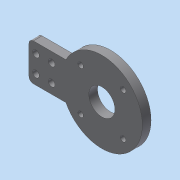
# Autodesk Inventor part: motormount3_B
Saved by Autodesk Inventor 2017 (Build 210142000, 142)
## iProperties
Created: 2015-12-27
Part Number: motormount3_B
Material: Generic
Document SubType Name: Modeling
Designer: JoshuaYuan
Density: 1 g/cm^3
Appearance: Default
Author: JoshuaYuan
Autodesk Inventor part; units mm, degrees
ref_plane "YZ Plane" through (0, 0, 0) normal (1, 0, 0) x (0, 1, 0)
ref_plane "XZ Plane" through (0, 0, 0) normal (0, 1, 0) x (-1, 0, 0)
ref_plane "XY Plane" through (0, 0, 0) normal (0, 0, 1) x (1, 0, 0)
sketch "Sketch1" plane through (0, 0, 0) normal (0, 0, 1) x (1, 0, 0)
  line L0 (-17.3159, 0) -> (99.2924, 0) projected
  line L1 (0, -41.3) -> (0, 41.3) projected
  circle A0 centre (53.1341, 0) radius 29.5
  line L2 (26.924, 13.5382) -> (3.175, 13.5382)
  line L3 (0, 10.3632) -> (0, -10.3632)
  line L4 (3.175, -13.5382) -> (26.924, -13.5382)
  arc A1 (3.175, 13.5382) -> (0, 10.3632) centre (3.175, 10.3632) ccw
  arc A2 (0, -10.3632) -> (3.175, -13.5382) centre (3.175, -10.3632) ccw
  circle A3 centre (5.08, 6.35) radius 2.413
  circle A4 centre (16.51, 6.35) radius 2.413
  circle A5 centre (5.08, -6.35) radius 2.413
  circle A6 centre (16.51, -6.35) radius 2.413
  circle A7 centre (37.6341, 15.5) radius 2
  circle A8 centre (68.6341, 15.5) radius 2
  circle A9 centre (68.6341, -15.5) radius 2
  circle A10 centre (37.6341, -15.5) radius 2
  line L5 (73.9937, 20.8597) -> (32.2744, -20.8597) construction
  line L6 (32.2744, 20.8597) -> (73.9937, -20.8597) construction
  circle A11 centre (53.1341, 0) radius 9.525
  point P0 (0, 0)
  point P1 (0, -13.5382)
  dimension "d0" = 59
  dimension "d2" = 3.175
  dimension "d9" = 20.7264
  dimension "d10" = 4.826
  dimension "d15" = 11.43
  dimension "d18" = 12.7
  dimension "d21" = 4
  dimension "d23" = 4
  dimension "d24" = 4
  dimension "d25" = 4
  dimension "d26" = 45
  dimension "d45" = 19.05
  dimension "d48" = 31
  dimension "d49" = 31
  dimension "d50" = 31
  dimension "d51" = 5.08
  dimension "d52" = 26.924
  dimension "d53" = 15.5
  constraints: 12 centre point, 10 end point, 10 point on circle, 7 point on line, 4 midpoint, 4 tangent, 3 perpendicular, 2 horizontal, 1 coincident, 1 collinear, 1 equal radius, 1 parallel, 1 vertical, 7 other
  measures "d0" diameter of A0
  measures "d2" radius of A1
  measures "d9" distance of L3.start L3.end
  measures "d10" diameter of A3
  measures "d15" distance of A3.centre A4.centre
  measures "d18" distance of A3.centre A5.centre
  measures "d21" diameter of A7
  measures "d23" diameter of A8
  measures "d24" diameter of A9
  measures "d25" diameter of A10
  measures "d26" angle of L0 L5
  measures "d45" diameter of A11
  measures "d48" distance of A10.centre A7.centre
  measures "d49" distance of A8.centre A7.centre
  measures "d50" distance of A9.centre A8.centre
  measures "d51" distance from line of L3 A5.centre
  measures "d52" distance from line of L4.end L3
  measures "d53" horizontal distance of A0.centre A9.centre
extrude "plate" add sketch "Sketch1" along normal blind 6.35
extrude "motor hole" cut sketch "Sketch1" along normal blind 25.4 contours A11 L0 | L0 A11
equation "\"d21\" = bolt_holes"
equation "\"d23\" = bolt_holes"
equation "\"d24\" = bolt_holes"
equation "\"d25\" = bolt_holes"
equation "\"bolt_holes\" = 4"
body "Solid1"
